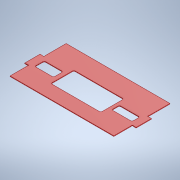
# Autodesk Inventor part: Cockpit_back_frame_cloth
Saved by Autodesk Inventor 2020 (Build 240168000, 168)
## iProperties
Part Number: Cockpit_back_frame_cloth
Material: PET プラスチック
Document SubType Name: Modeling
Designer: Masato Kubotera
Density: 1.541 g/cm^3
Appearance: 滑らか - 赤
Description: PP T0.75
Mass: 8.71306 g
Surface Area: 156.509 cm^2
Volume: 5.65416 cm^3
Author: Masato Kubotera
Autodesk Inventor part; units mm, degrees
ref_plane "YZ Plane" through (0, 0, 0) normal (1, 0, 0) x (0, 1, 0)
ref_plane "XZ Plane" through (0, 0, 0) normal (0, 1, 0) x (-1, 0, 0)
ref_plane "XY Plane" through (0, 0, 0) normal (0, 0, 1) x (1, 0, 0)
derived "Cockpit_back_frame.ipt"
sketch "スケッチ2" plane through (0, 0, 0) normal (0, 1, 0) x (-1, 0, 0)
  line L0 (-23.5, -22.5) -> (-28.5, -27.5)
  line L1 (-28.5, -27.5) -> (-28.5, -91)
  line L2 (-28.5, -91) -> (-23.5, -96)
  line L3 (-23.5, -96) -> (34.25, -96)
  line L4 (36.25, -98) -> (36.25, -131)
  line L5 (36.25, -131) -> (41.25, -136)
  line L6 (41.25, -136) -> (86.5, -136)
  line L7 (91.5, -131) -> (91.5, -20)
  line L8 (91.5, -20) -> (89, -17.5)
  line L9 (89, -17.5) -> (83.25, -17.5)
  line L10 (83.25, -17.5) -> (83.25, -21.0151)
  line L11 (81.7651, -22.5) -> (76.9849, -22.5)
  line L12 (75.5, -21.0151) -> (75.5, -17.5)
  line L13 (75.5, -17.5) -> (67.5, -17.5)
  line L14 (67.5, -17.5) -> (67.5, -21.0151)
  line L15 (66.0151, -22.5) -> (-23.5, -22.5)
  line L16 (-25.25, -25) -> (-20.25, -25) construction
  line L17 (-20.25, -25) -> (-20.25, -93.5) construction
  line L18 (-20.25, -93.5) -> (-25.25, -93.5) construction
  line L19 (-25.25, -93.5) -> (-25.25, -25) construction
  line L20 (-26, -25) -> (-25.25, -25) construction
  line L21 (-25.25, -93.5) -> (-26, -93.5) construction
  line L22 (-26, -93.5) -> (-26, -25) construction
  line L23 (-20.25, -93.5) -> (83.25, -93.5) construction
  line L24 (-20.25, -88.5) -> (83.25, -88.5) construction
  line L25 (83.25, -22.5) -> (83.25, -90.5) construction
  line L26 (83.25, -90.5) -> (88.25, -90.5) construction
  line L27 (88.25, -90.5) -> (88.25, -22.5) construction
  line L28 (83.25, -88.5) -> (83.25, -93.5) construction
  line L29 (83.25, -91) -> (88.25, -91) construction
  line L30 (88.25, -91) -> (88.25, -133.5) construction
  line L31 (83.25, -91) -> (83.25, -133.5) construction
  line L32 (83.25, -133.5) -> (88.25, -133.5) construction
  line L33 (38.75, -133.5) -> (38.75, -128.5) construction
  line L34 (38.75, -128.5) -> (38.75, -93.5) construction
  line L35 (43.75, -93.5) -> (43.75, -128.5) construction
  line L36 (38.75, -128.5) -> (43.75, -128.5) construction
  line L37 (41.25, -128.5) -> (41.25, -93.5) construction
  line L38 (38.75, -128.5) -> (82.1145, -128.5) construction
  line L39 (82.1145, -128.5) -> (82.1145, -133.5) construction
  line L40 (82.1145, -133.5) -> (38.75, -133.5) construction
  line L41 (38.75, -131) -> (82.1145, -131) construction
  line L42 (85.75, -91) -> (85.75, -133.5) construction
  circle A0 centre (85.75, -131) radius 2
  arc A1 (83.25, -128.5) -> (88.25, -128.5) centre (85.75, -131) ccw construction
  line L43 (83.25, -91) -> (-20.25, -91) construction
  line L44 (41.25, -111) -> (43.75, -111) construction
  line L45 (60.4322, -128.5) -> (60.4322, -131) construction
  line L46 (41.2, -115.5651) -> (41.2, -106.4349)
  line L47 (43.8, -107.05) -> (43.8, -114.95)
  line L48 (43.8, -117.05) -> (41.2, -104.95) construction
  line L49 (41.2, -117.05) -> (43.8, -104.95) construction
  line L50 (56.4822, -128.45) -> (64.3822, -128.45)
  line L51 (64.9973, -131.05) -> (55.8672, -131.05)
  line L52 (54.3822, -128.45) -> (66.4822, -131.05) construction
  line L53 (66.4822, -128.45) -> (54.3822, -131.05) construction
  line L54 (41.25, -105) -> (43.75, -105) construction
  line L55 (41.25, -117) -> (43.75, -117) construction
  arc A2 (42.6849, -104.95) -> (41.2, -106.4349) centre (41.9425, -105.6925) ccw
  arc A3 (43.8, -107.05) -> (43.8, -104.95) centre (43.8, -106) ccw
  arc A4 (41.2, -115.5651) -> (42.6849, -117.05) centre (41.9425, -116.3075) ccw
  arc A5 (43.8, -117.05) -> (43.8, -114.95) centre (43.8, -116) ccw
  line L56 (54.4322, -131) -> (54.4322, -128.5) construction
  line L57 (66.4322, -128.5) -> (66.4322, -131) construction
  arc A6 (54.3822, -129.5651) -> (55.8672, -131.05) centre (55.1247, -130.3075) ccw
  arc A7 (56.4822, -128.45) -> (54.3822, -128.45) centre (55.4322, -128.45) ccw
  arc A8 (64.9973, -131.05) -> (66.4822, -129.5651) centre (65.7398, -130.3075) ccw
  arc A9 (66.4822, -128.45) -> (64.3822, -128.45) centre (65.4322, -128.45) ccw
  line L58 (54.3822, -129.5651) -> (54.3822, -128.45)
  line L59 (66.4822, -128.45) -> (66.4822, -129.5651)
  line L60 (42.6849, -104.95) -> (43.8, -104.95)
  line L61 (43.8, -117.05) -> (42.6849, -117.05)
  circle A10 centre (48.4322, -131) radius 1.6
  line L62 (88.25, -22.5) -> (88.25, -17.5) construction
  line L63 (89, -17.5) -> (89, -90.5) construction
  line L64 (89, -90.5) -> (88.25, -90.5) construction
  line L65 (-13.5, -82.5) -> (-13.5, -61)
  arc A11 (-13.5, -82.5) -> (-11.5, -84.5) centre (-11.5, -82.5) ccw
  line L66 (45.5, -84.5) -> (-11.5, -84.5)
  arc A12 (45.5, -84.5) -> (47.5, -82.5) centre (45.5, -82.5) ccw
  line L67 (47.5, -61) -> (47.5, -82.5)
  arc A13 (47.5, -61) -> (45.5, -59) centre (45.5, -61) ccw
  line L68 (-11.5, -59) -> (45.5, -59)
  arc A14 (-11.5, -59) -> (-13.5, -61) centre (-11.5, -61) ccw
  line L69 (31.5, -88.5) -> (31.5, -91) construction
  line L70 (85.75, -22.5) -> (85.75, -90.5) construction
  circle A15 centre (85.75, -34) radius 1.6
  circle A16 centre (85.75, -34) radius 3
  circle A17 centre (85.75, -79) radius 1.6
  circle A18 centre (85.75, -79) radius 3
  line L71 (88.25, -22.5) -> (83.25, -22.5) construction
  arc A19 (88.25, -91) -> (83.25, -91) centre (85.75, -131) ccw construction
  circle A20 centre (48.4322, -131) radius 3
  circle A21 centre (41.25, -99) radius 1.6
  circle A22 centre (41.25, -99) radius 3
  line L72 (6.5, -88.5) -> (6.5, -91) construction
  line L73 (56.5, -88.5) -> (56.5, -91) construction
  line L74 (55.0651, -91.05) -> (7.9349, -91.05)
  line L75 (6.45, -89.5651) -> (6.45, -88.45)
  line L76 (8.55, -88.45) -> (54.45, -88.45)
  line L77 (56.55, -88.45) -> (56.55, -89.5651)
  line L78 (56.55, -91.05) -> (6.45, -88.45) construction
  line L79 (6.45, -91.05) -> (56.55, -88.45) construction
  arc A23 (8.55, -88.45) -> (6.45, -88.45) centre (7.5, -88.45) ccw
  arc A24 (6.45, -89.5651) -> (7.9349, -91.05) centre (7.1925, -90.3075) ccw
  arc A25 (56.55, -88.45) -> (54.45, -88.45) centre (55.5, -88.45) ccw
  arc A26 (55.0651, -91.05) -> (56.55, -89.5651) centre (55.8075, -90.3075) ccw
  line L80 (-20.25, -41) -> (83.25, -41) construction
  line L81 (83.25, -36) -> (-20.25, -36) construction
  line L82 (-20.25, -36) -> (-20.25, -41) construction
  line L83 (-20.25, -38.5) -> (83.25, -38.5) construction
  line L84 (31.5, -41) -> (31.5, -36) construction
  line L85 (55.0651, -35.95) -> (7.9349, -35.95)
  line L86 (7.9349, -41.05) -> (55.0651, -41.05)
  line L87 (56.55, -35.95) -> (6.45, -41.05) construction
  line L88 (6.45, -35.95) -> (55.5877, -40.952) construction
  arc A27 (7.9349, -35.95) -> (6.45, -37.4349) centre (7.1925, -36.6925) ccw
  arc A28 (6.45, -39.5651) -> (7.9349, -41.05) centre (7.1925, -40.3075) ccw
  arc A29 (56.55, -37.4349) -> (55.0651, -35.95) centre (55.8075, -36.6925) ccw
  arc A30 (55.0651, -41.05) -> (56.55, -39.5651) centre (55.8075, -40.3075) ccw
  line L89 (6.5, -41) -> (6.5, -36) construction
  line L90 (56.5, -36) -> (56.5, -41) construction
  line L91 (6.45, -37.4349) -> (6.45, -39.5651)
  line L92 (56.55, -39.5651) -> (56.55, -37.4349)
  circle A31 centre (-1, -38.5) radius 1.6
  circle A32 centre (-1, -38.5) radius 3
  circle A33 centre (64, -38.5) radius 1.6
  circle A34 centre (64, -38.5) radius 3
  line L93 (-25.25, -49.25) -> (-26, -49.25) construction
  line L94 (-25.25, -69.25) -> (-26, -69.25) construction
  line L95 (-26, -59.25) -> (-25.25, -59.25) construction
  line L96 (-22.75, -25) -> (-22.75, -93.5) construction
  arc A35 (66.0151, -22.5) -> (67.5, -21.0151) centre (66.7575, -21.7575) ccw
  arc A36 (75.5, -21.0151) -> (76.9849, -22.5) centre (76.2425, -21.7575) ccw
  line L97 (59.75, -22.5) -> (59.75, -32.5) construction
  line L98 (59.75, -32.5) -> (83.25, -32.5) construction
  line L99 (83.25, -32.5) -> (83.25, -22.5) construction
  line L100 (71.5, -17.5) -> (71.5, -32.5) construction
  line L101 (63.5, -22.5) -> (63.5, -17.5) construction
  line L102 (79.5, -22.5) -> (79.5, -17.5) construction
  circle A37 centre (-22.75, -31.75) radius 1.6
  circle A38 centre (-22.75, -31.75) radius 3
  circle A39 centre (-22.75, -86.75) radius 1.6
  circle A40 centre (-22.75, -86.75) radius 3
  line L103 (67.5, -22.5) -> (75.5, -22.5)
  line L104 (88.25, -17.5) -> (52.5, -17.5) construction
  line L105 (52.5, -17.5) -> (52.5, -22.5) construction
  circle A41 centre (85.75, -98.5) radius 1.475
  circle A42 centre (85.75, -103.5) radius 1.475
  circle A43 centre (85.75, -108.5) radius 1.475
  line L106 (48.25, -93.5) -> (78.75, -93.5)
  line L107 (80.75, -95.5) -> (80.75, -124)
  line L108 (78.75, -126) -> (48.25, -126)
  line L109 (46.25, -124) -> (46.25, -95.5)
  arc A44 (48.25, -93.5) -> (46.25, -95.5) centre (48.25, -95.5) ccw
  arc A45 (46.25, -124) -> (48.25, -126) centre (48.25, -124) ccw
  arc A46 (78.75, -126) -> (80.75, -124) centre (78.75, -124) ccw
  arc A47 (80.75, -95.5) -> (78.75, -93.5) centre (78.75, -95.5) ccw
  arc A48 (36.25, -98) -> (34.25, -96) centre (34.25, -98) ccw
  circle A49 centre (-13.5, -55) radius 1.75
  circle A50 centre (-13.5, -55) radius 2
  line L110 (77.85, -78.65) -> (68.65, -78.65) construction
  line L111 (68.65, -78.65) -> (68.65, -64.85) construction
  line L112 (68.65, -64.85) -> (77.85, -64.85) construction
  line L113 (77.85, -64.85) -> (77.85, -78.65) construction
  line L114 (77.85, -78.65) -> (68.65, -64.85) construction
  line L115 (68.65, -78.65) -> (77.85, -64.85) construction
  line L116 (67.95, -64.2) -> (78.55, -64.2) construction
  line L117 (78.55, -64.2) -> (78.55, -79.3) construction
  line L118 (78.55, -79.3) -> (67.95, -79.3) construction
  line L119 (67.95, -79.3) -> (67.95, -64.2) construction
  line L120 (67.95, -64.2) -> (78.55, -79.3) construction
  line L121 (78.55, -64.2) -> (67.95, -79.3) construction
  line L122 (69.3849, -64.15) -> (77.1151, -64.15)
  line L123 (78.6, -65.6349) -> (78.6, -77.8651)
  line L124 (78.6, -79.35) -> (67.9, -64.15) construction
  line L125 (67.9, -79.35) -> (78.6, -64.15) construction
  line L126 (77.9, -78.7) -> (68.6, -64.8) construction
  line L127 (68.6, -78.7) -> (77.9, -64.8) construction
  arc A51 (69.3849, -64.15) -> (67.9, -65.6349) centre (68.6425, -64.8925) ccw
  arc A52 (70.0849, -64.8) -> (68.6, -66.2849) centre (69.3425, -65.5425) ccw
  line L128 (67.9, -71.75) -> (78.6, -71.75) construction
  line L129 (73.25, -64.15) -> (73.25, -78.7063) construction
  arc A53 (78.6, -65.6349) -> (77.1151, -64.15) centre (77.8575, -64.8925) ccw
  arc A54 (77.9, -66.2849) -> (76.4151, -64.8) centre (77.1575, -65.5425) ccw
  arc A55 (67.9, -77.8651) -> (69.3849, -79.35) centre (68.6425, -78.6075) ccw
  arc A56 (68.6, -77.2151) -> (70.0849, -78.7) centre (69.3425, -77.9575) ccw
  arc A57 (77.1151, -79.35) -> (78.6, -77.8651) centre (77.8575, -78.6075) ccw
  arc A58 (76.4151, -78.7) -> (77.9, -77.2151) centre (77.1575, -77.9575) ccw
  line L130 (70.0849, -64.8) -> (76.4151, -64.8)
  line L131 (77.9, -66.2849) -> (77.9, -77.2151)
  line L132 (67.9, -77.8651) -> (67.9, -65.6349)
  line L133 (68.6, -77.2151) -> (68.6, -66.2849)
  line L134 (76.4151, -78.7) -> (70.0849, -78.7)
  line L135 (77.1151, -79.35) -> (69.3849, -79.35)
  line L136 (-13.5, -71.75) -> (47.5, -71.75) construction
  line L137 (85.75, -56.5) -> (88.25, -56.5) construction
  line L138 (89, -54) -> (88.25, -54) construction
  line L139 (85.7, -69.45) -> (85.7, -43.55)
  line L140 (88.2835, -71.3588) -> (85.7, -41.45) construction
  line L141 (85.7, -71.55) -> (88.3, -41.45) construction
  arc A59 (85.7, -41.45) -> (85.7, -43.55) centre (85.7, -42.5) ccw
  arc A60 (88.3, -42.9349) -> (86.8151, -41.45) centre (87.5575, -42.1925) ccw
  arc A61 (85.7, -69.45) -> (85.7, -71.55) centre (85.7, -70.5) ccw
  arc A62 (86.8151, -71.55) -> (88.3, -70.0651) centre (87.5575, -70.8075) ccw
  line L142 (85.75, -41.5) -> (88.25, -41.5) construction
  line L143 (85.75, -71.5) -> (88.25, -71.5) construction
  arc A63 (89.25, -47.1801) -> (88.3, -46.1348) centre (88.2, -47.1801) ccw
  line L144 (89.25, -47.1801) -> (89.25, -65.8199)
  line L145 (88.25, -46.5) -> (89, -46.5) construction
  line L146 (88.25, -66.5) -> (89, -66.5) construction
  arc A64 (88.3, -66.8652) -> (89.25, -65.8199) centre (88.2, -65.8199) ccw
  line L147 (88.3, -42.9349) -> (88.3, -46.1348)
  line L148 (88.3, -66.8652) -> (88.3, -70.0651)
  line L149 (86.8151, -71.55) -> (85.7, -71.55)
  line L150 (85.7, -41.45) -> (86.8151, -41.45)
  line L151 (86.5, -136) -> (91.5, -131)
  arc A65 (81.7651, -22.5) -> (83.25, -21.0151) centre (82.5075, -21.7575) ccw
  circle A66 centre (85.75, -93.5) radius 2
  circle A67 centre (85.75, -93.5) radius 4 construction
  arc A68 (-24.15, -49.25) -> (-26.25, -49.25) centre (-25.2, -49.25) ccw
  line L152 (-26, -49.25) -> (-26.25, -49.25) construction
  line L153 (-26.25, -49.25) -> (-26.25, -69.25)
  line L154 (-24.15, -49.25) -> (-24.15, -69.25)
  arc A69 (-26.25, -69.25) -> (-24.15, -69.25) centre (-25.2, -69.25) ccw
  point P0 (0, 0)
  point P1 (-25.7227, -96)
  point P2 (-23.5, -22.5)
  point P3 (42.5, -111)
  point P4 (60.4322, -129.75)
  point P5 (31.5, -89.75)
  point P6 (31.5, -38.5)
  point P7 (6.45, -41.05)
  point P8 (52.5, -22)
  point P9 (73.25, -71.75)
  point P10 (73.25, -71.75)
  point P11 (87, -56.5)
  dimension "d4" = 0.75
  measures "d4" distance of L63.end L26.end
sketch "スケッチ3" plane through (-88.25, 0, 0) normal (1, 0, 0) x (0, 1, 0)
  line L0 (-135, -22.5) -> (0, -22.5)
  line L1 (0, -22.5) -> (0, -40.0151)
  line L2 (0, -90.5) -> (-135, -90.5)
  line L3 (-135, -56.5) -> (0, -56.5) construction
  line L4 (-67.5, -22.5) -> (-67.5, -90.5) construction
  line L5 (1.4849, -41.5) -> (5, -41.5)
  line L6 (5, -41.5) -> (5, -71.5)
  line L7 (5, -71.5) -> (1.4849, -71.5)
  arc A0 (0, -40.0151) -> (1.4849, -41.5) centre (0.7425, -40.7575) ccw
  arc A1 (1.4849, -71.5) -> (0, -72.9849) centre (0.7425, -72.2425) ccw
  line L8 (0, -41.5) -> (0, -71.5)
  line L9 (0, -72.9849) -> (0, -90.5)
  line L10 (-135, -41.5) -> (-135, -71.5)
  line L11 (-135, -22.5) -> (-135, -40.0151)
  arc A2 (-136.4849, -41.5) -> (-135, -40.0151) centre (-135.7425, -40.7575) ccw
  line L12 (-136.4849, -41.5) -> (-140, -41.5)
  line L13 (-140, -41.5) -> (-140, -71.5)
  line L14 (-135, -72.9849) -> (-135, -90.5)
  arc A3 (-135, -72.9849) -> (-136.4849, -71.5) centre (-135.7425, -72.2425) ccw
  line L15 (-140, -71.5) -> (-136.4849, -71.5)
  line L16 (-98, -42.5) -> (-37, -42.5)
  line L17 (-35, -44.5) -> (-35, -70.5)
  line L18 (-37, -72.5) -> (-98, -72.5)
  line L19 (-100, -70.5) -> (-100, -44.5)
  arc A4 (-98, -42.5) -> (-100, -44.5) centre (-98, -44.5) ccw
  arc A5 (-100, -70.5) -> (-98, -72.5) centre (-98, -70.5) ccw
  arc A6 (-37, -72.5) -> (-35, -70.5) centre (-37, -70.5) ccw
  arc A7 (-35, -44.5) -> (-37, -42.5) centre (-37, -44.5) ccw
  line L20 (-125.25, -53.45) -> (-125.25, -61.55) construction
  line L21 (-117.5, -53.2) -> (-117.5, -61.8) construction
  line L22 (-109.5, -53.2) -> (-125.5, -53.2)
  line L23 (-125.5, -61.8) -> (-109.5, -53.2) construction
  line L24 (-109.5, -61.8) -> (-125.5, -53.2) construction
  line L25 (-109.75, -53.45) -> (-125.25, -53.45) construction
  line L26 (-109.75, -61.55) -> (-109.75, -53.45) construction
  line L27 (-109.75, -53.45) -> (-125.25, -61.55) construction
  circle A8 centre (-107.5, -57.5) radius 1.35
  circle A9 centre (-107.5, -57.5) radius 2.25 construction
  line L28 (-125.25, -53.45) -> (-109.75, -61.55) construction
  circle A10 centre (-127.5, -57.5) radius 1.35
  line L29 (-109.5, -61.8) -> (-109.5, -53.2)
  line L30 (-125.5, -61.8) -> (-109.5, -61.8)
  line L31 (-125.25, -61.55) -> (-109.75, -61.55) construction
  line L32 (-107.5, -57.5) -> (-127.5, -57.5) construction
  line L33 (-125.5, -53.2) -> (-125.5, -61.8)
  line L34 (-28.75, -62.75) -> (-6.25, -62.75) construction
  line L35 (-17.5, -52.25) -> (-17.5, -62.75) construction
  line L36 (-6.25, -52.25) -> (-28.75, -52.25) construction
  line L37 (-28.75, -52.25) -> (-6.25, -62.75) construction
  line L38 (-28.75, -62.75) -> (-6.25, -52.25) construction
  line L39 (-29, -63) -> (-6, -63)
  line L40 (-6, -52) -> (-29, -52)
  line L41 (-29, -52) -> (-6, -63) construction
  line L42 (-29, -63) -> (-6, -52) construction
  line L43 (-30.5, -57.5) -> (-4.5, -57.5) construction
  arc A11 (-7.4849, -63) -> (-6, -61.5151) centre (-6.7425, -62.2575) ccw
  line L44 (-6.25, -62.75) -> (-6.25, -52.25) construction
  line L45 (-6, -63) -> (-6, -52)
  arc A12 (-6, -53.4849) -> (-7.4849, -52) centre (-6.7425, -52.7425) ccw
  circle A13 centre (-4.5, -57.5) radius 0.8
  line L46 (-28.75, -52.25) -> (-28.75, -62.75) construction
  line L47 (-29, -52) -> (-29, -63)
  arc A14 (-27.5151, -52) -> (-29, -53.4849) centre (-28.2575, -52.7425) ccw
  arc A15 (-29, -61.5151) -> (-27.5151, -63) centre (-28.2575, -62.2575) ccw
  circle A16 centre (-30.5, -57.5) radius 0.8
  arc A17 (-109.5, -54.6849) -> (-110.9849, -53.2) centre (-110.2425, -53.9425) ccw
  arc A18 (-110.9849, -61.8) -> (-109.5, -60.3151) centre (-110.2425, -61.0575) ccw
  arc A19 (-125.5, -60.3151) -> (-124.0151, -61.8) centre (-124.7575, -61.0575) ccw
  arc A20 (-124.0151, -53.2) -> (-125.5, -54.6849) centre (-124.7575, -53.9425) ccw
  line L48 (-130, -29.5) -> (-130, -46.45)
  line L49 (-128, -48.45) -> (-107, -48.45)
  line L50 (-128, -27.5) -> (-107, -27.5)
  line L51 (-105, -29.5) -> (-105, -46.45)
  line L52 (-28, -27.5) -> (-7, -27.5)
  line L53 (-5, -29.5) -> (-5, -45.25)
  line L54 (-7, -47.25) -> (-28, -47.25)
  line L55 (-30, -45.25) -> (-30, -29.5)
  line L56 (-98, -27.5) -> (-37, -27.5)
  line L57 (-35, -29.5) -> (-35, -38)
  line L58 (-37, -40) -> (-98, -40)
  line L59 (-100, -38) -> (-100, -29.5)
  line L60 (-128, -66.55) -> (-107, -66.55)
  line L61 (-7, -67.75) -> (-28, -67.75)
  line L62 (-37, -75) -> (-98, -75)
  line L63 (-98, -85.5) -> (-37, -85.5)
  line L64 (-128, -85.5) -> (-107, -85.5)
  line L65 (-28, -85.5) -> (-7, -85.5)
  line L66 (-130, -68.55) -> (-130, -83.5)
  line L67 (-105, -68.55) -> (-105, -83.5)
  line L68 (-100, -83.5) -> (-100, -77)
  line L69 (-35, -77) -> (-35, -83.5)
  line L70 (-30, -83.5) -> (-30, -69.75)
  line L71 (-5, -69.75) -> (-5, -83.5)
  arc A21 (-128, -27.5) -> (-130, -29.5) centre (-128, -29.5) ccw
  arc A22 (-130, -46.45) -> (-128, -48.45) centre (-128, -46.45) ccw
  arc A23 (-107, -48.45) -> (-105, -46.45) centre (-107, -46.45) ccw
  arc A24 (-105, -29.5) -> (-107, -27.5) centre (-107, -29.5) ccw
  arc A25 (-98, -27.5) -> (-100, -29.5) centre (-98, -29.5) ccw
  arc A26 (-100, -38) -> (-98, -40) centre (-98, -38) ccw
  arc A27 (-37, -40) -> (-35, -38) centre (-37, -38) ccw
  arc A28 (-35, -29.5) -> (-37, -27.5) centre (-37, -29.5) ccw
  arc A29 (-28, -27.5) -> (-30, -29.5) centre (-28, -29.5) ccw
  arc A30 (-5, -29.5) -> (-7, -27.5) centre (-7, -29.5) ccw
  arc A31 (-7, -47.25) -> (-5, -45.25) centre (-7, -45.25) ccw
  arc A32 (-30, -45.25) -> (-28, -47.25) centre (-28, -45.25) ccw
  arc A33 (-28, -67.75) -> (-30, -69.75) centre (-28, -69.75) ccw
  arc A34 (-30, -83.5) -> (-28, -85.5) centre (-28, -83.5) ccw
  arc A35 (-7, -85.5) -> (-5, -83.5) centre (-7, -83.5) ccw
  arc A36 (-5, -69.75) -> (-7, -67.75) centre (-7, -69.75) ccw
  arc A37 (-37, -85.5) -> (-35, -83.5) centre (-37, -83.5) ccw
  arc A38 (-35, -77) -> (-37, -75) centre (-37, -77) ccw
  arc A39 (-100, -83.5) -> (-98, -85.5) centre (-98, -83.5) ccw
  arc A40 (-98, -75) -> (-100, -77) centre (-98, -77) ccw
  arc A41 (-107, -85.5) -> (-105, -83.5) centre (-107, -83.5) ccw
  arc A42 (-105, -68.55) -> (-107, -66.55) centre (-107, -68.55) ccw
  arc A43 (-128, -66.55) -> (-130, -68.55) centre (-128, -68.55) ccw
  arc A44 (-130, -83.5) -> (-128, -85.5) centre (-128, -83.5) ccw
  point P0 (0, 0)
  point P1 (-135, -71.5)
  point P2 (0, -90.5)
  point P3 (0, -71.5)
  point P4 (0, -41.5)
  point P5 (-67.5, -42.5)
  point P6 (-117.5, -57.5)
  point P7 (-117.5, -57.5)
  point P8 (-17.5, -57.5)
  point P9 (-17.5, -57.5)
  point P10 (-125, -54.6849)
  point P11 (-123.5151, -53.2)
  point P12 (-110, -60.3151)
  point P13 (-111.4849, -61.8)
  point P14 (-123.5151, -61.8)
  point P15 (-125, -60.3151)
  point P16 (-27.5151, -63)
  point P17 (-7.4849, -52)
  point P18 (-6, -53.4849)
  point P19 (-6, -61.5151)
  point P20 (-7.4849, -63)
  point P21 (-100, -57.5)
  point P22 (-130, -27.5)
  point P23 (-130, -48.45)
  point P24 (-105, -27.5)
  point P25 (-105, -48.45)
  point P26 (-30, -27.5)
  point P27 (-5, -47.25)
  point P28 (-5, -27.5)
  point P29 (-30, -47.25)
  point P30 (-100, -27.5)
  point P31 (-35, -40)
  point P32 (-35, -27.5)
  point P33 (-100, -40)
  point P34 (-130, -66.55)
  point P35 (-105, -66.55)
  point P36 (-5, -67.75)
  point P37 (-30, -67.75)
  point P38 (-35, -75)
  point P39 (-100, -75)
  point P40 (-100, -85.5)
  point P41 (-35, -85.5)
  point P42 (-130, -85.5)
  point P43 (-105, -85.5)
  point P44 (-30, -85.5)
  point P45 (-5, -85.5)
  point P46 (-135, -71.5)
  point P47 (-125.5, -54.6849)
  point P48 (-124.0151, -53.2)
  point P49 (-109.5, -60.3151)
  point P50 (-110.9849, -61.8)
  point P51 (-124.0151, -61.8)
  point P52 (-125.5, -60.3151)
  point P53 (-27.5151, -63)
  point P54 (-7.4849, -52)
  point P55 (-6, -53.4849)
  point P56 (-6, -61.5151)
  point P57 (-7.4849, -63)
ref_plane "作業平面1" through (-88.25, -135, -22.5) normal (-1, 0, 0) x (0, 1, 0)
sketch "スケッチ4" plane through (-88.25, -135, -22.5) normal (-1, 0, 0) x (0, 1, 0)
  line L0 (136.4849, 24) -> (140, 24)
  arc A0 (136.4849, 24) -> (135, 22.5151) centre (135.7425, 23.2575) ccw
  line L1 (135, 108.5) -> (135, -2.5) construction
  line L2 (140, 19) -> (140, 49) construction
  line L3 (136.4849, 44) -> (140, 44)
  arc A1 (135, 45.4849) -> (136.4849, 44) centre (135.7425, 44.7425) ccw
  line L4 (140, 44) -> (140, 24)
  line L5 (135, -5) -> (135, 22.5151)
  line L6 (135, 45.4849) -> (135, 68)
  line L7 (135, 68) -> (0, 68) projected
  line L8 (135, -5) -> (0, -5)
  line L9 (67.5, -5) -> (67.5, 68) construction
  line L10 (-1.4849, 24) -> (-5, 24)
  arc A2 (0, 22.5151) -> (-1.4849, 24) centre (-0.7425, 23.2575) ccw
  arc A3 (-1.4849, 44) -> (0, 45.4849) centre (-0.7425, 44.7425) ccw
  line L11 (-1.4849, 44) -> (-5, 44)
  line L12 (-5, 44) -> (-5, 24)
  line L13 (0, -5) -> (0, 22.5151)
  line L14 (0, 45.4849) -> (0, 68)
  arc A4 (100, 48) -> (98, 50) centre (98, 48) ccw projected
  line L15 (100, 22) -> (100, 48) projected
  arc A5 (98, 20) -> (100, 22) centre (98, 22) ccw projected
  line L16 (37, 20) -> (98, 20) projected
  line L17 (98, 50) -> (37, 50) projected
  line L18 (35, 48) -> (35, 22) projected
  arc A6 (35, 22) -> (37, 20) centre (37, 22) ccw projected
  arc A7 (37, 50) -> (35, 48) centre (37, 48) ccw projected
  line L19 (28.75, 40.05) -> (6.25, 40.05)
  line L20 (4.25, 38.05) -> (4.25, 31.95)
  line L21 (6.25, 29.95) -> (28.75, 29.95)
  line L22 (30.75, 31.95) -> (30.75, 38.05)
  line L23 (30.75, 40.05) -> (4.25, 29.95) construction
  line L24 (4.25, 40.05) -> (30.75, 29.95) construction
  line L25 (9.75, 39.05) -> (25.25, 39.05) construction
  circle A8 centre (27.5, 35) radius 2.25 construction
  arc A9 (30.75, 38.05) -> (28.75, 40.05) centre (28.75, 38.05) ccw
  arc A10 (6.25, 40.05) -> (4.25, 38.05) centre (6.25, 38.05) ccw
  arc A11 (4.25, 31.95) -> (6.25, 29.95) centre (6.25, 31.95) ccw
  arc A12 (28.75, 29.95) -> (30.75, 31.95) centre (28.75, 31.95) ccw
  line L26 (128.75, 40.25) -> (128.75, 29.75) construction
  line L27 (106.25, 40.25) -> (128.75, 40.25) construction
  line L28 (107.25, 28.75) -> (127.75, 28.75)
  line L29 (129.75, 30.75) -> (129.75, 39.25)
  line L30 (127.75, 41.25) -> (107.25, 41.25)
  line L31 (105.25, 39.25) -> (105.25, 30.75)
  line L32 (105.25, 28.75) -> (129.75, 41.25) construction
  line L33 (129.75, 28.75) -> (105.25, 41.25) construction
  arc A13 (129.75, 39.25) -> (127.75, 41.25) centre (127.75, 39.25) ccw
  arc A14 (107.25, 41.25) -> (105.25, 39.25) centre (107.25, 39.25) ccw
  arc A15 (105.25, 30.75) -> (107.25, 28.75) centre (107.25, 30.75) ccw
  arc A16 (127.75, 28.75) -> (129.75, 30.75) centre (127.75, 30.75) ccw
  line L34 (135, 44) -> (135, 24)
  line L35 (0, 44) -> (0, 24)
  point P0 (135, -22.5)
  point P1 (135, 34)
  point P2 (67.5, 0)
  point P3 (25.5, 37.8151)
  point P4 (17.5, 35)
  point P5 (117.5, 35)
  dimension "d1" = 1.05
  dimension "d5" = 1.05
  dimension "d8" = 1
  dimension "d9" = 1
  dimension "d10" = 2
  dimension "d11" = 2
  dimension "d12" = 1
  dimension "d13" = 1
  constraints: 52 end point, 28 point on circle, 22 point on line, 16 tangent, 12 centre point, 9 symmetric about line, 6 equal radius, 5 midpoint, 5 parallel, 4 perpendicular, 4 vertical, 3 horizontal, 1 coincident, 6 other
  measures "d1" radius of A0
  measures "d5" radius of A1
  measures "d8" distance edge to line of A8 L22
  measures "d9" distance between parallel lines of L19 L25
  measures "d10" radius of A9
  measures "d11" radius of A13
  measures "d12" distance between parallel lines of L29 L26
  measures "d13" distance between parallel lines of L30 L27
extrude "押し出し1" add sketch "スケッチ4" along normal blind 0.75
equation "\"d5\" = d1"
equation "\"d9\" = d8"
equation "\"d12\" = d8"
equation "\"d13\" = d12"
equation "\"d2\" = d4"
